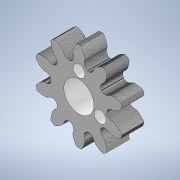
# Autodesk Inventor part: ギア_歯数20モジュール2
Saved by Autodesk Inventor 2021 (Build 250183000, 183)
## iProperties
Created: 2022-02-11
Part Number: ギア_歯数20モジュール2
Material: 一般
Document SubType Name: Modeling
Designer: hirohumi
Density: 1 g/cm^3
Appearance: 既定
Autodesk Inventor part; units mm, degrees
ref_plane "YZ Plane" through (0, 0, 0) normal (1, 0, 0) x (0, 1, 0)
ref_plane "XZ Plane" through (0, 0, 0) normal (0, 1, 0) x (-1, 0, 0)
ref_plane "XY Plane" through (0, 0, 0) normal (0, 0, 1) x (1, 0, 0)
sketch "スケッチ1" plane through (0, 0, 0) normal (0, 0, 1) x (1, 0, 0)
  point P0 (0, 0)
sketch "0" plane through (0, 0, 0) normal (0, 0, 1) x (1, 0, 0)
  circle A0 centre (0, 0) radius 10 construction
  line L0 (-12, 0) -> (12, 0) construction
  line L1 (0, -12) -> (0, 12) construction
  line L2 (7.5, 0) -> (7.5, 0.0193)
  line L3 (7.5, 0.0193) -> (7.4999, 0.0386)
  line L4 (7.4999, 0.0386) -> (7.4998, 0.0579)
  line L5 (7.4998, 0.0579) -> (7.4996, 0.0772)
  line L6 (7.4996, 0.0772) -> (7.4994, 0.0965)
  line L7 (7.4994, 0.0965) -> (7.5117, 0.2593)
  line L8 (7.5117, 0.2593) -> (7.5389, 0.3899)
  line L9 (7.5389, 0.3899) -> (7.5773, 0.4987)
  line L10 (7.5773, 0.4987) -> (7.6247, 0.6017)
  line L11 (7.6247, 0.6017) -> (7.6809, 0.6927)
  line L12 (7.6809, 0.6927) -> (7.7446, 0.7812)
  line L13 (7.7446, 0.7812) -> (7.8163, 0.8592)
  line L14 (7.8163, 0.8592) -> (7.8947, 0.9351)
  line L15 (7.8947, 0.9351) -> (7.9805, 1.002)
  line L16 (7.9805, 1.002) -> (8.073, 1.0648)
  line L17 (8.073, 1.0648) -> (8.1722, 1.1216)
  line L18 (8.1722, 1.1216) -> (8.2785, 1.1696)
  line L19 (8.2785, 1.1696) -> (8.3906, 1.2165)
  line L20 (8.3906, 1.2165) -> (8.5096, 1.2534)
  line L21 (8.5096, 1.2534) -> (8.635, 1.2841)
  line L22 (8.635, 1.2841) -> (8.7662, 1.3116)
  line L23 (8.7662, 1.3116) -> (8.9041, 1.3288)
  line L24 (8.9041, 1.3288) -> (9.0482, 1.3379)
  line L25 (9.0482, 1.3379) -> (9.1975, 1.3458)
  line L26 (9.1975, 1.3458) -> (9.3531, 1.3425)
  line L27 (9.3531, 1.3425) -> (9.4765, 1.3804)
  line L28 (9.4765, 1.3804) -> (9.5985, 1.4278)
  line L29 (9.5985, 1.4278) -> (9.7192, 1.4825)
  line L30 (9.7192, 1.4825) -> (9.8388, 1.5436)
  line L31 (9.8388, 1.5436) -> (9.9573, 1.6103)
  line L32 (9.9573, 1.6103) -> (10.0748, 1.6824)
  line L33 (10.0748, 1.6824) -> (10.1911, 1.7595)
  line L34 (10.1911, 1.7595) -> (10.3062, 1.8413)
  line L35 (10.3062, 1.8413) -> (10.4201, 1.9276)
  line L36 (10.4201, 1.9276) -> (10.5328, 2.0184)
  line L37 (10.5328, 2.0184) -> (10.6443, 2.1134)
  line L38 (10.6443, 2.1134) -> (10.7543, 2.2126)
  line L39 (10.7543, 2.2126) -> (10.863, 2.3158)
  line L40 (10.863, 2.3158) -> (10.9703, 2.423)
  line L41 (10.9703, 2.423) -> (11.0761, 2.534)
  line L42 (11.0761, 2.534) -> (11.1803, 2.6489)
  line L43 (11.1803, 2.6489) -> (11.2829, 2.7675)
  line L44 (11.2829, 2.7675) -> (11.3839, 2.8897)
  line L45 (11.3839, 2.8897) -> (11.4831, 3.0156)
  line L46 (11.4831, 3.0156) -> (11.5805, 3.145)
  line L47 (11.5805, 3.145) -> (11.5492, 3.2583)
  line L48 (11.5492, 3.2583) -> (11.5167, 3.3713)
  line L49 (11.5167, 3.3713) -> (11.4831, 3.4839)
  line L50 (11.4831, 3.4839) -> (11.4485, 3.5962)
  line L51 (11.4485, 3.5962) -> (11.4127, 3.7082)
  line L52 (7.5, 0) -> (7.5, -0.0193)
  line L53 (7.5, -0.0193) -> (7.4999, -0.0386)
  line L54 (7.4999, -0.0386) -> (7.4998, -0.0579)
  line L55 (7.4998, -0.0579) -> (7.4996, -0.0772)
  line L56 (7.4996, -0.0772) -> (7.4994, -0.0965)
  line L57 (7.4994, -0.0965) -> (7.5117, -0.2593)
  line L58 (7.5117, -0.2593) -> (7.5389, -0.3899)
  line L59 (7.5389, -0.3899) -> (7.5773, -0.4987)
  line L60 (7.5773, -0.4987) -> (7.6247, -0.6017)
  line L61 (7.6247, -0.6017) -> (7.6809, -0.6927)
  line L62 (7.6809, -0.6927) -> (7.7446, -0.7812)
  line L63 (7.7446, -0.7812) -> (7.8163, -0.8592)
  line L64 (7.8163, -0.8592) -> (7.8947, -0.9351)
  line L65 (7.8947, -0.9351) -> (7.9805, -1.002)
  line L66 (7.9805, -1.002) -> (8.073, -1.0648)
  line L67 (8.073, -1.0648) -> (8.1722, -1.1216)
  line L68 (8.1722, -1.1216) -> (8.2785, -1.1696)
  line L69 (8.2785, -1.1696) -> (8.3906, -1.2165)
  line L70 (8.3906, -1.2165) -> (8.5096, -1.2534)
  line L71 (8.5096, -1.2534) -> (8.635, -1.2841)
  line L72 (8.635, -1.2841) -> (8.7662, -1.3116)
  line L73 (8.7662, -1.3116) -> (8.9041, -1.3288)
  line L74 (8.9041, -1.3288) -> (9.0482, -1.3379)
  line L75 (9.0482, -1.3379) -> (9.1975, -1.3458)
  line L76 (9.1975, -1.3458) -> (9.3531, -1.3425)
  line L77 (9.3531, -1.3425) -> (9.4765, -1.3804)
  line L78 (9.4765, -1.3804) -> (9.5985, -1.4278)
  line L79 (9.5985, -1.4278) -> (9.7192, -1.4825)
  line L80 (9.7192, -1.4825) -> (9.8388, -1.5436)
  line L81 (9.8388, -1.5436) -> (9.9573, -1.6103)
  line L82 (9.9573, -1.6103) -> (10.0748, -1.6824)
  line L83 (10.0748, -1.6824) -> (10.1911, -1.7595)
  line L84 (10.1911, -1.7595) -> (10.3062, -1.8413)
  line L85 (10.3062, -1.8413) -> (10.4201, -1.9276)
  line L86 (10.4201, -1.9276) -> (10.5328, -2.0184)
  line L87 (10.5328, -2.0184) -> (10.6443, -2.1134)
  line L88 (10.6443, -2.1134) -> (10.7543, -2.2126)
  line L89 (10.7543, -2.2126) -> (10.863, -2.3158)
  line L90 (10.863, -2.3158) -> (10.9703, -2.423)
  line L91 (10.9703, -2.423) -> (11.0761, -2.534)
  line L92 (11.0761, -2.534) -> (11.1803, -2.6489)
  line L93 (11.1803, -2.6489) -> (11.2829, -2.7675)
  line L94 (11.2829, -2.7675) -> (11.3839, -2.8897)
  line L95 (11.3839, -2.8897) -> (11.4831, -3.0156)
  line L96 (11.4831, -3.0156) -> (11.5805, -3.145)
  line L97 (11.5805, -3.145) -> (11.5492, -3.2583)
  line L98 (11.5492, -3.2583) -> (11.5167, -3.3713)
  line L99 (11.5167, -3.3713) -> (11.4831, -3.4839)
  line L100 (11.4831, -3.4839) -> (11.4485, -3.5962)
  line L101 (11.4485, -3.5962) -> (11.4127, -3.7082)
  line L102 (11.4127, 3.7082) -> (0, 0)
  line L103 (0, 0) -> (11.4127, -3.7082)
  constraints: 208 end point, 50 symmetric about line, 1 centre point, 1 perpendicular, 1 point on line
extrude "押し出し1" add sketch "0" along normal blind 6
pattern_circular "円形状パターン1" count 10 over 360 about axis through (0, 0, 0) along (0, 0, 1) of "押し出し1"
sketch "スケッチ3" plane through (0, 0, 6) normal (0, 0, 1) x (1, 0, 0)
  circle A0 centre (0, 0) radius 4.05
  circle A1 centre (0, 6) radius 1.6
  circle A2 centre (5.7063, -1.8541) radius 1.6
  line L0 (0, 6) -> (0, 0) construction
  line L1 (0, 0) -> (5.7063, -1.8541) construction
  dimension "d5" = 8.1
  dimension "d6" = 3.2
  dimension "d7" = 3.2
  dimension "d9" = 6
  dimension "d10" = 108
  dimension "d11" = 6
  constraints: 4 end point, 3 centre point, 1 coincident, 1 vertical
  measures "d5" diameter of A0
  measures "d6" diameter of A1
  measures "d7" diameter of A2
  measures "d9" distance of point (0, 0) L0.start
  measures "d10" angle of L1 L0
  measures "d11" distance of L1.end point (0, 0)
extrude "押し出し2" cut sketch "スケッチ3" against normal through all
